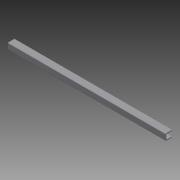
# Autodesk Inventor part: c-channel
Saved by Autodesk Inventor 2015 SP1 (Build 190203100, 203)
## iProperties
Created: 2015-01-13
Part Number: c-channel
Material: Generic
Document SubType Name: Modeling
Designer: Jarod
Density: 1 g/cm^3
Appearance: Default
Author: Jarod
Autodesk Inventor part; units mm, degrees
ref_plane "YZ Plane" through (0, 0, 0) normal (1, 0, 0) x (0, 1, 0)
ref_plane "XZ Plane" through (0, 0, 0) normal (0, 1, 0) x (-1, 0, 0)
ref_plane "XY Plane" through (0, 0, 0) normal (0, 0, 1) x (1, 0, 0)
sketch "Sketch1" plane through (0, 0, 0) normal (1, 0, 0) x (0, 1, 0)
  line L0 (0, 0) -> (0, 22.225)
  line L1 (3.175, 25.4) -> (22.225, 25.4)
  line L2 (25.4, 22.225) -> (25.4, 0)
  line L3 (22.225, 0) -> (22.225, 22.225)
  line L4 (22.225, 22.225) -> (3.175, 22.225)
  line L5 (3.175, 22.225) -> (3.175, 0)
  line L6 (0, 0) -> (3.175, 0)
  line L7 (22.225, 0) -> (25.4, 0)
  arc A0 (3.175, 25.4) -> (0, 22.225) centre (3.175, 22.225) ccw
  arc A1 (25.4, 22.225) -> (22.225, 25.4) centre (22.225, 22.225) ccw
  point P0 (0, 25.4)
  point P1 (25.4, 25.4)
  dimension "d0" = 25.4
  dimension "d2" = 25.4
  dimension "d3" = 90
  dimension "d4" = 25.4
  dimension "d5" = 90
  dimension "d6" = 3.175
  dimension "d7" = 3.175
  constraints: 16 end point, 4 perpendicular, 4 point on circle, 4 point on line, 4 tangent, 2 centre point, 1 collinear, 1 equal radius, 1 horizontal, 1 vertical, 2 other
  measures "d0" distance of L0.start point (0, 25.4)
  measures "d2" distance of point (0, 25.4) point (25.4, 25.4)
  measures "d3" angle of L0 L1
  measures "d4" distance of point (25.4, 25.4) L2.end
  measures "d5" angle of L1 L2
  measures "d6" distance between parallel lines of L1 L4
  measures "d7" radius of A0
extrude "Extrusion1" add sketch "Sketch1" along normal blind 685.8
sketch "Sketch2" plane through (0, 25.4, 22.225) normal (0, 1, 0) x (1, 0, 0)
  line L0 (0, 0) -> (0, 22.225) projected
  line L1 (0, 0) -> (685.8, 0) projected
  line L2 (685.8, 22.225) -> (685.8, 0) projected
  line L3 (0, 22.225) -> (685.8, 22.225) projected
  point P0 (12.7, 9.525)
  dimension "d10" = 12.7
  dimension "d11" = 12.7
  measures "d10" distance from line of L0 point (12.7, 9.525)
  measures "d11" distance from line of L3 point (12.7, 9.525)
hole "Hole1" at (12.7, 25.4, 12.7) direction (0, -1, 0) diameter 6.35 end through all
pattern_linear "Rectangular Pattern1" count 27 spacing 25.4 along (1, 0, 0) of "Hole1"
body "Solid1"
